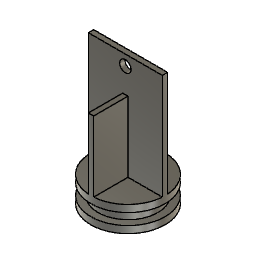
dpv2_plunger (Autodesk Fusion 360 design; units mm, degrees)
Autodesk Fusion 360 part; units mm, degrees
sketch "スケッチ1" plane through (0, 0, 0) normal (0, 0, 1) x (1, 0, 0)
  circle A0 centre (0, 0) radius 10.55
  dimension "d1" = 21.1
  constraint coincident A0.centre origin
  measures "d1" diameter of A0
extrude "押し出し1" add sketch "スケッチ1" along normal blind 2
sketch "スケッチ2" plane through (0, 0, 2) normal (0, 0, 1) x (-1, 0, 0)
  circle A0 centre (0, 0) radius 10.55
  circle A1 centre (0, 0) radius 8.5
  dimension "d4" = 17
  constraint coincident A0.centre A1.centre
  measures "d4" diameter of A1
extrude "押し出し2" add sketch "スケッチ2" along normal blind 3.2 contours A1
sketch "スケッチ3" plane through (0, 0, 5.2) normal (0, 0, 1) x (-1, 0, 0)
  circle A0 centre (0, 0) radius 8.5
  circle A1 centre (0, 0) radius 10.55
extrude "押し出し3" add sketch "スケッチ3" along normal blind 2 contours A0 | A1
sketch "スケッチ4" plane through (0, 0, 7.2) normal (0, 0, 1) x (-1, 0, 0)
  line L0 (10.5233, -0.75) -> (-10.5233, -0.75)
  line L1 (10.5233, 0.75) -> (-10.5233, 0.75)
  circle A0 centre (0, 0) radius 10.55
  dimension "d24" = 0.75
  dimension "d25" = 0.75
  constraint horizontal L0
  constraint parallel L0 L1
  constraint coincident L0.end A0
  constraint coincident L1.end A0
  constraint coincident L0.start A0
  constraint coincident L1.start A0
  measures "d24" distance of A0.centre L0
  measures "d25" distance of A0.centre L1
extrude "押し出し7" add sketch "スケッチ4" along normal blind 30 contours L0 L1 A0
sketch "スケッチ5" plane through (0, -0.75, 0) normal (0, -1, 0) x (1, 0, 0)
  line L0 (-10.4732, 7.2) -> (10.4732, 7.2)
  line L1 (10.5, 7.2) -> (10.5, 37.2)
  line L2 (10.5, 37.2) -> (-10.5, 37.2)
  line L3 (-10.5, 37.2) -> (-10.5, 7.2)
  circle A0 centre (0, 34.2) radius 1.625
  line L4 (0, 34.2) -> (0, 37.2) construction
  line L5 (10.4732, 7.2) -> (10.5, 7.2)
  line L6 (-10.5, 7.2) -> (-10.4732, 7.2)
  line L7 (-10.5233, 7.2) -> (10.5233, 7.2)
  line L8 (10.5233, 7.2) -> (10.5233, 37.2)
  line L9 (10.5233, 37.2) -> (-10.5233, 37.2)
  line L10 (-10.5233, 37.2) -> (-10.5233, 7.2)
  dimension "d13" = 3.25
  dimension "d14" = 3
  constraint coincident A0.centre L4.start
  constraint midpoint L2 L4.end
  constraint perpendicular L2 L4
  measures "d13" diameter of A0
  measures "d14" distance of L2 A0.centre
extrude "押し出し8" cut sketch "スケッチ5" against normal up to surface (1.5 mm away) contours A0
sketch "スケッチ8" plane through (0, 0, 7.2) normal (0, 0, 1) x (-1, 0, 0)
  line L0 (-10.5233, 0.75) -> (10.5233, 0.75)
  arc A0 (10.5233, 0.75) -> (-10.5233, 0.75) centre (0, 0) ccw
  line L1 (0.75, -10.5233) -> (0.75, 10.5233)
  line L2 (-0.75, -10.5233) -> (-0.75, 10.5233)
  arc A1 (-10.5233, -0.75) -> (10.5233, -0.75) centre (0, 0) ccw
  dimension "d30" = 0.75
  dimension "d31" = 0.75
  constraint vertical L1
  constraint vertical L2
  constraint coincident L1.start A1
  constraint coincident L2.start A1
  constraint coincident A0 L2.end
  constraint coincident A0 L1.end
  measures "d30" distance of A0.centre L2
  measures "d31" distance of A0.centre L1
extrude "押し出し9" add sketch "スケッチ8" along normal blind 20 contours L0 A0 L1 L2 | L0 L1 L2 A1
